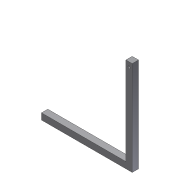
# Autodesk Inventor part: Stinger
Saved by Autodesk Inventor 2012 (Build 160160000, 160)
## iProperties
Created: 2012-03-04
Part Number: Stinger
Material: Default
Document SubType Name: Modeling
Designer: JesseK
Density: 1 g/cm^3
Author: JesseK
Autodesk Inventor part; units mm, degrees
ref_plane "YZ Plane" through (0, 0, 0) normal (1, 0, 0) x (0, 1, 0)
ref_plane "XZ Plane" through (0, 0, 0) normal (0, 1, 0) x (-1, 0, 0)
ref_plane "XY Plane" through (0, 0, 0) normal (0, 0, 1) x (1, 0, 0)
sketch "Sketch1" plane through (0, 0, 0) normal (0, 0, 1) x (1, 0, 0)
  circle A0 centre (0, 0) radius 4.7625
  line L0 (12.7, -419.1) -> (12.7, 38.1)
  line L1 (12.7, 38.1) -> (-12.7, 38.1)
  line L2 (-12.7, 38.1) -> (-12.7, -419.1)
  line L3 (-12.7, -419.1) -> (12.7, -419.1)
  dimension "d0" = 9.525
  dimension "d2" = 12.7
  dimension "d3" = 38.1
  dimension "d4" = 457.2
  constraints: 8 end point, 2 perpendicular, 1 centre point, 1 coincident, 1 horizontal, 1 parallel
  measures "d0" diameter of A0
  measures "d2" distance from line of L2 A0.centre
  measures "d3" distance from line of A0.centre L1
  measures "d4" distance of L0.start L0.end
extrude "Extrusion1" add sketch "Sketch1" along normal blind 25.4
sketch "Sketch2" plane through (0, 0, 25.4) normal (0, 0, 1) x (1, 0, 0)
  line L0 (12.7, -419.1) -> (-12.7, -419.1) projected
  line L1 (12.7, 38.1) -> (12.7, -419.1) projected
  circle A0 centre (0, -406.4) radius 3.175
  dimension "d7" = 12.7
  dimension "d8" = 12.7
  dimension "d9" = 6.35
  constraints: 1 centre point
  measures "d7" distance from line of L1 A0.centre
  measures "d8" distance from line of L0 A0.centre
  measures "d9" diameter of A0
extrude "Extrusion2" cut sketch "Sketch2" against normal up to next
body "Solid1"
